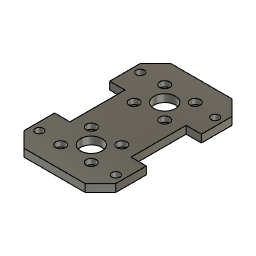
X#XZ_connector (Autodesk Fusion 360 design; units mm, degrees)
Autodesk Fusion 360 part; units mm, degrees
note: some values were not read from the file. Set by a fixed rule: which sketch regions a step uses.
sketch "Sketch1" plane through (0, 0, 0) normal (0, 0, 1) x (1, 0, 0)
  line L0 (0, 0) -> (40, 0)
  line L1 (40, 0) -> (40, 96)
  line L2 (40, 96) -> (0, 96)
  line L3 (0, 96) -> (0, 0)
  line L4 (20, 0) -> (20, 15)
  line L5 (20, 96) -> (20, 81)
  circle A0 centre (20, 81) radius 2.65
  circle A1 centre (20, 15) radius 2.65
  dimension "d1" = 40
  dimension "d2" = 96
  dimension "d3" = 15
  dimension "d4" = 5.3
  dimension "d5" = 5.3
  constraint horizontal L0
  constraint vertical L1
  constraint horizontal L2
  constraint vertical L3
  constraint coincident L0.start L3.end
  constraint midpoint L0 L4.start
  constraint perpendicular L0 L4
  constraint midpoint L2 L5.start
  constraint perpendicular L2 L5
  constraint coincident L5.end A0.centre
  constraint coincident L4.end A1.centre
  measures "d1" distance of L0.start L0.end
  measures "d2" distance of L0.start L2.end
  measures "d3" distance of L5.start L5.end
  measures "d4" diameter of A0
  measures "d5" diameter of A1
extrude "Extrude1" add sketch "Sketch1" along normal blind 5
sketch "Sketch2" plane through (0, 0, 5) normal (0, 0, 1) x (-1, 0, 0)
  circle A0 centre (-20, -15) radius 2.65
  circle A1 centre (-20, -81) radius 2.65
  line L0 (0, -96) -> (0, 0)
  line L1 (0, 0) -> (-40, 0)
  line L2 (-40, 0) -> (-40, -96)
  line L3 (-40, -96) -> (0, -96)
  line L4 (0, -48) -> (-40, -48)
  line L5 (-20, -46.5) -> (-20, -1.5)
  line L6 (-20, -34) -> (-30, -34)
  line L7 (-30, -34) -> (-30, -14)
  line L8 (-30, -14) -> (-10, -14)
  line L9 (-10, -14) -> (-10, -34)
  line L10 (-10, -34) -> (-20, -34)
  line L11 (-20, -49.5) -> (-20, -94.5)
  line L12 (-20, -62) -> (-30, -62)
  line L13 (-30, -62) -> (-30, -82)
  line L14 (-30, -82) -> (-10, -82)
  line L15 (-10, -82) -> (-10, -62)
  line L16 (-10, -62) -> (-20, -62)
  circle A2 centre (-30, -14) radius 1.55
  circle A3 centre (-10, -14) radius 1.55
  circle A4 centre (-10, -34) radius 1.55
  circle A5 centre (-30, -34) radius 1.55
  circle A6 centre (-30, -62) radius 1.55
  circle A7 centre (-10, -62) radius 1.55
  circle A8 centre (-10, -82) radius 1.55
  circle A9 centre (-30, -82) radius 1.55
  dimension "d12" = 45
  dimension "d15" = 45
  dimension "d16" = 3.1
  dimension "d17" = 3.1
  dimension "d18" = 3.1
  dimension "d19" = 3.1
  dimension "d20" = 3.1
  dimension "d21" = 3.1
  dimension "d22" = 3.1
  dimension "d23" = 3.1
  constraint midpoint L0 L4.start
  constraint midpoint L2 L4.end
  constraint coincident L5 L6.start
  constraint perpendicular L6 L7
  constraint perpendicular L5 L8
  constraint perpendicular L8 L9
  constraint vertical L11
  constraint coincident L11 L12.start
  constraint perpendicular L12 L13
  constraint perpendicular L11 L14
  constraint perpendicular L14 L15
  constraint perpendicular L11 L16
  constraint coincident L7.end L8.start
  constraint coincident L8.end L9.start
  constraint coincident L9.end L10.start
  constraint coincident L6.end L7.start
  constraint coincident L12.end L13.start
  constraint coincident L15.end L16.start
  constraint coincident L14.end L15.start
  constraint coincident L13.end L14.start
  measures "d12" distance of L5.start L5.end
  measures "d15" distance of L11.start L11.end
  measures "d16" diameter of A2
  measures "d17" diameter of A3
  measures "d18" diameter of A4
  measures "d19" diameter of A5
  measures "d20" diameter of A6
  measures "d21" diameter of A7
  measures "d22" diameter of A8
  measures "d23" diameter of A9
extrude "Extrude2" cut sketch "Sketch2" against normal blind 5 contours L8 L9 A3 | L8 L9 A3 | L7 L8 A2 | L7 L8 A2 | L6 L7 A5 | L6 L7 A5 | L9 L10 A4 | L9 L10 A4 | L14 L15 A8 | L14 L15 A8 | L13 L14 A9 | L13 L14 A9 | L12 L13 A6 | L12 L13 A6 | L15 L16 A7 | L15 L16 A7
sketch "Sketch3" plane through (0, 0, 5) normal (0, 0, 1) x (-1, 0, 0)
  circle A0 centre (-30, -34) radius 1.55
  circle A1 centre (-10, -82) radius 1.55
  circle A2 centre (-10, -62) radius 1.55
  circle A3 centre (-30, -14) radius 1.55
  circle A4 centre (-10, -34) radius 1.55
  circle A5 centre (-30, -82) radius 1.55
  circle A6 centre (-10, -14) radius 1.55
  circle A7 centre (-30, -62) radius 1.55
  circle A8 centre (-20, -15) radius 2.65
  circle A9 centre (-20, -81) radius 2.65
  line L0 (0, -96) -> (0, 0)
  line L1 (0, 0) -> (-40, 0)
  line L2 (-40, 0) -> (-40, -96)
  line L3 (-40, -96) -> (0, -96)
  circle A10 centre (-20, -15) radius 2.65
  circle A11 centre (-20, -81) radius 2.65
  constraint concentric A8 A10
  constraint concentric A9 A11
extrude "Extrude3" add sketch "Sketch3" against normal blind 5 contours A8 A10 | A9 A11
sketch "Sketch4" plane through (0, 0, 0) normal (0, 0, 1) x (1, 0, 0)
  line L0 (-10, 0) -> (-10, 30)
  line L1 (-10, 30) -> (0, 30)
  line L2 (-5, 0) -> (-5, 15)
  circle A0 centre (-5, 15) radius 2.6
  line L3 (40, 0) -> (50, 0)
  line L4 (50, 0) -> (50, 30)
  line L5 (50, 30) -> (40, 30)
  line L6 (40, 30) -> (45, 15)
  circle A1 centre (45, 15) radius 2.6
  line L7 (40, 96) -> (50, 96)
  line L8 (50, 96) -> (50, 66)
  line L9 (50, 66) -> (40, 66)
  line L10 (40, 66) -> (45, 80)
  circle A2 centre (45, 80) radius 2.6
  line L11 (0, 96) -> (-10, 96)
  line L12 (-10, 96) -> (-10, 66)
  line L13 (-10, 66) -> (0, 66)
  line L14 (0, 66) -> (-5, 81)
  circle A3 centre (-5, 81) radius 2.6
  line L15 (-10, 0) -> (-9, 0)
  line L16 (-9, 0) -> (0, 0)
  line L17 (0, 0) -> (0, 30)
  line L18 (40, 30) -> (40, 0)
  line L19 (0, 66) -> (0, 96)
  line L20 (40, 96) -> (40, 66)
  dimension "d28" = 5.2
  dimension "d29" = 5.2
  dimension "d30" = 5.2
  dimension "d31" = 5.2
  constraint perpendicular L0 L1
  constraint coincident L2.end A0.centre
  constraint horizontal L3
  constraint perpendicular L3 L4
  constraint perpendicular L4 L5
  constraint coincident L6.end A1.centre
  constraint horizontal L7
  constraint perpendicular L7 L8
  constraint perpendicular L8 L9
  constraint coincident L10.end A2.centre
  constraint horizontal L11
  constraint perpendicular L11 L12
  constraint perpendicular L12 L13
  constraint coincident L14.end A3.centre
  constraint perpendicular L0 L15
  constraint coincident L16.end L17.start
  constraint perpendicular L0 L16
  constraint perpendicular L1 L17
  constraint perpendicular L3 L18
  constraint perpendicular L11 L19
  constraint perpendicular L11 L20
  measures "d28" diameter of A0
  measures "d29" diameter of A1
  measures "d30" diameter of A2
  measures "d31" diameter of A3
extrude "Extrude4" add sketch "Sketch4" along normal blind 5
chamfer "Chamfer1" distance 10 angle 45 1 edges at (-10, 0, 2.5)
chamfer "Chamfer2" distance 10 angle 45 1 edges at (50, 0, 2.5)
chamfer "Chamfer3" distance 10 angle 45 1 edges at (-10, 96, 2.5)
chamfer "Chamfer4" distance 10 angle 45 1 edges at (50, 96, 2.5)
sketch "Sketch5" plane through (0, 0, 5) normal (0, 0, 1) x (-1, 0, 0)
  circle A0 centre (-45, -80) radius 2.6
  circle A1 centre (-45, -15) radius 2.6
  circle A2 centre (5, -81) radius 2.6
  circle A3 centre (5, -15) radius 2.6
  circle A4 centre (-30, -34) radius 1.55
  circle A5 centre (-10, -82) radius 1.55
  circle A6 centre (-10, -62) radius 1.55
  circle A7 centre (-30, -14) radius 1.55
  circle A8 centre (-10, -34) radius 1.55
  circle A9 centre (-30, -82) radius 1.55
  circle A10 centre (-10, -14) radius 1.55
  circle A11 centre (-30, -62) radius 1.55
  line L0 (-50, -86) -> (-40, -96)
  line L1 (-40, -96) -> (0, -96)
  line L2 (0, -96) -> (10, -86)
  line L3 (10, -86) -> (10, -66)
  line L4 (10, -66) -> (0, -66)
  line L5 (0, -66) -> (0, -30)
  line L6 (0, -30) -> (10, -30)
  line L7 (10, -30) -> (10, -10)
  line L8 (10, -10) -> (0, 0)
  line L9 (0, 0) -> (-40, 0)
  line L10 (-40, 0) -> (-50, -10)
  line L11 (-50, -10) -> (-50, -30)
  line L12 (-50, -30) -> (-40, -30)
  line L13 (-40, -30) -> (-40, -66)
  line L14 (-40, -66) -> (-50, -66)
  line L15 (-50, -66) -> (-50, -86)
  line L16 (-10, -62) -> (-30, -82)
  line L17 (-10, -14) -> (-30, -34)
  circle A12 centre (-20, -24) radius 7
  circle A13 centre (-20, -72) radius 7
  dimension "d38" = 14
  dimension "d39" = 14
  constraint coincident A6.centre L16.start
  constraint coincident A9.centre L16.end
  constraint coincident A10.centre L17.start
  constraint coincident A4.centre L17.end
  constraint midpoint L17 A12.centre
  constraint midpoint L16 A13.centre
  measures "d38" diameter of A12
  measures "d39" diameter of A13
extrude "Extrude5" cut sketch "Sketch5" against normal blind 5 contours L16 A13 | L16 A13 | L17 A12 | L17 A12
sketch "Sketch6" plane through (0, 0, 5) normal (0, 0, 1) x (-1, 0, 0)
  circle A0 centre (-20, -24) radius 7
  circle A1 centre (-20, -72) radius 7
  circle A2 centre (-45, -80) radius 2.6
  circle A3 centre (-45, -15) radius 2.6
  circle A4 centre (5, -81) radius 2.6
  circle A5 centre (5, -15) radius 2.6
  circle A6 centre (-30, -34) radius 1.55
  circle A7 centre (-10, -82) radius 1.55
  circle A8 centre (-10, -62) radius 1.55
  circle A9 centre (-30, -14) radius 1.55
  circle A10 centre (-10, -34) radius 1.55
  circle A11 centre (-30, -82) radius 1.55
  circle A12 centre (-10, -14) radius 1.55
  circle A13 centre (-30, -62) radius 1.55
  line L0 (-50, -86) -> (-40, -96)
  line L1 (-40, -96) -> (0, -96)
  line L2 (0, -96) -> (10, -86)
  line L3 (10, -86) -> (10, -66)
  line L4 (10, -66) -> (0, -66)
  line L5 (0, -66) -> (0, -30)
  line L6 (0, -30) -> (10, -30)
  line L7 (10, -30) -> (10, -10)
  line L8 (10, -10) -> (0, 0)
  line L9 (0, 0) -> (-40, 0)
  line L10 (-40, 0) -> (-50, -10)
  line L11 (-50, -10) -> (-50, -30)
  line L12 (-50, -30) -> (-40, -30)
  line L13 (-40, -30) -> (-40, -66)
  line L14 (-40, -66) -> (-50, -66)
  line L15 (-50, -66) -> (-50, -86)
  circle A14 centre (-10, -82) radius 3.25
  circle A15 centre (-30, -82) radius 3.25
  circle A16 centre (-30, -62) radius 3.25
  circle A17 centre (-10, -62) radius 3.25
  circle A18 centre (-10, -34) radius 3.25
  circle A19 centre (-30, -34) radius 3.25
  circle A20 centre (-30, -14) radius 3.25
  circle A21 centre (-10, -14) radius 3.25
  dimension "d42" = 6.5
  dimension "d43" = 6.5
  dimension "d44" = 6.5
  dimension "d45" = 6.5
  dimension "d46" = 6.5
  dimension "d47" = 6.5
  dimension "d48" = 6.5
  dimension "d49" = 6.5
  constraint concentric A7 A14
  constraint concentric A11 A15
  constraint concentric A13 A16
  constraint concentric A8 A17
  constraint concentric A10 A18
  constraint concentric A6 A19
  constraint concentric A9 A20
  constraint concentric A12 A21
  measures "d42" diameter of A14
  measures "d43" diameter of A15
  measures "d44" diameter of A16
  measures "d45" diameter of A17
  measures "d46" diameter of A18
  measures "d47" diameter of A19
  measures "d48" diameter of A20
  measures "d49" diameter of A21
extrude "Extrude6" cut sketch "Sketch6" against normal blind 3.5 contours A14 | A15 | A16 | A17 | A18 | A19 | A20 | A21
